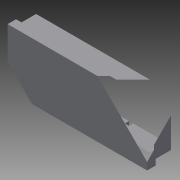
# Autodesk Inventor part: NoiseSourceWell
Saved by Autodesk Inventor 2014 (Build 180170000, 170)
## iProperties
Created: 2015-11-06
Part Number: NoiseSourceWell
Material: Generic
Document SubType Name: Modeling
Designer: Owner
Density: 1 g/cm^3
Appearance: Default
Author: Owner
Autodesk Inventor part; units mm, degrees
ref_plane "YZ Plane" through (0, 0, 0) normal (1, 0, 0) x (0, 1, 0)
ref_plane "XZ Plane" through (0, 0, 0) normal (0, 1, 0) x (-1, 0, 0)
ref_plane "XY Plane" through (0, 0, 0) normal (0, 0, 1) x (1, 0, 0)
sketch "Sketch1" plane through (0, 0, 0) normal (0, 0, 1) x (1, 0, 0)
  line L0 (-53.3723, 20.7143) -> (51.8738, 20.7143)
  line L1 (51.8738, 20.7143) -> (51.8738, -22.3009)
  line L2 (51.8738, -22.3009) -> (-53.3723, -22.3009)
  line L3 (-53.3723, -22.3009) -> (-53.3723, 20.7143)
  point P0 (0, 0)
  constraints: 8 end point, 2 parallel, 1 horizontal, 1 perpendicular
extrude "Extrusion1" add sketch "Sketch1" along normal blind 6.35
sketch "Sketch2" plane through (0, 0, 0) normal (0, 0, -1) x (-1, 0, 0)
  line L0 (-51.8738, 20.7143) -> (53.3723, 20.7143)
  line L1 (53.3723, 20.7143) -> (53.3723, -22.3009)
  line L2 (53.3723, -22.3009) -> (-51.8738, -22.3009)
  line L3 (-51.8738, -22.3009) -> (-51.8738, 20.7143)
  line L4 (-47.5602, 15.8741) -> (47.7562, 15.8741)
  line L5 (47.7562, 15.8741) -> (47.7562, -15.8759)
  line L6 (47.7562, -15.8759) -> (-47.5602, -15.8759)
  line L7 (-47.5602, -15.8759) -> (-47.5602, 15.8741)
  line L8 (-50.7352, 19.0491) -> (50.9312, 19.0491)
  line L9 (50.9312, 19.0491) -> (50.9312, -19.0509)
  line L10 (50.9312, -19.0509) -> (-50.7352, -19.0509)
  line L11 (-50.7352, -19.0509) -> (-50.7352, 19.0491)
  line L12 (53.3723, -22.3009) -> (53.3723, 20.7143) projected
  line L13 (-47.5602, -9.4351) -> (-33.4749, -9.4351)
  line L14 (-33.4749, -9.4351) -> (-29.5119, -13.2742)
  line L15 (-29.5119, -13.2742) -> (-8.1285, -13.2742)
  line L16 (-8.1285, -13.2742) -> (-5.4429, -15.8759)
  point P0 (0, 0)
  dimension "d6" = 3.175
  dimension "d7" = 3.175
  dimension "d8" = 31.75
  dimension "d9" = 3.175
  dimension "d10" = 3.175
  constraints: 32 end point, 8 parallel, 4 perpendicular, 3 horizontal, 2 point on line
  measures "d6" distance between parallel lines of L4 L8
  measures "d7" distance between parallel lines of L10 L6
  measures "d8" distance between parallel lines of L4 L6
  measures "d9" distance between parallel lines of L11 L7
  measures "d10" distance between parallel lines of L9 L5
extrude "Extrusion2" add sketch "Sketch2" along normal blind 12.7 contours L13 L14 L15 L16 L6 L7 | L8 L9 L10 L11
sketch "Sketch4" plane through (0, 0, -12.7) normal (0, 0, -1) x (-1, 0, 0)
  line L0 (47.7562, -15.8759) -> (-5.4429, -15.8759) projected
  line L1 (27.7708, -15.8759) -> (39.4699, -15.8759)
  line L2 (39.4699, -15.8759) -> (39.4699, -22.2961)
  line L3 (39.4699, -22.2961) -> (27.7708, -22.2961)
  line L4 (27.7708, -22.2961) -> (27.7708, -15.8759)
  line L5 (-11.0473, -12.4096) -> (-8.1285, -12.4096)
  line L6 (-8.1285, -12.4096) -> (-8.1285, -20.4181)
  line L7 (-8.1285, -20.4181) -> (-11.0473, -20.4181)
  line L8 (-11.0473, -20.4181) -> (-11.0473, -12.4096)
  point P0 (-47.5602, -15.8759)
  point P1 (0, 0)
  constraints: 16 end point, 4 parallel, 2 horizontal, 2 perpendicular, 1 point on line
extrude "Extrusion4" cut sketch "Sketch4" against normal blind 3.175
body "Solid1"
